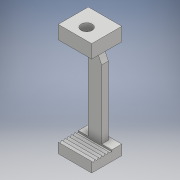
# Autodesk Inventor part: gravity-clamp-base5x5mm-part1-narrowTOP
Saved by Autodesk Inventor 2017 (Build 210142000, 142)
## iProperties
Created: 2021-08-04
Part Number: gravity-clamp-base5x5mm-part1-narrowTOP
Material: Generic
Document SubType Name: Modeling
Designer: Nikita
Density: 1 g/cm^3
Appearance: Default
Author: Nikita
Autodesk Inventor part; units mm, degrees
ref_plane "YZ Plane" through (0, 0, 0) normal (1, 0, 0) x (0, 1, 0)
ref_plane "XZ Plane" through (0, 0, 0) normal (0, 1, 0) x (-1, 0, 0)
ref_plane "XY Plane" through (0, 0, 0) normal (0, 0, 1) x (1, 0, 0)
sketch "Sketch1" plane through (0, 0, 0) normal (0, 0, 1) x (1, 0, 0)
  line L0 (0, 0) -> (10, 0)
  line L1 (10, 0) -> (10, 9)
  line L2 (10, 9) -> (0, 9)
  line L3 (0, 9) -> (0, 0)
  point P0 (5, 9)
  dimension "d0" = 10
  dimension "d1" = 9
  constraints: 8 end point, 2 parallel, 1 horizontal, 1 midpoint, 1 perpendicular
  measures "d0" distance of L2.end L1.end
  measures "d1" distance of L1.end L0.end
extrude "Extrusion1" add sketch "Sketch1" along normal blind 3
sketch "Sketch2" plane through (0, 0, 3) normal (0, 0, 1) x (1, 0, 0)
  line L0 (10, 9) -> (0, 9) projected
  circle A0 centre (5, 7) radius 1
  line L1 (0, 9) -> (0, 0) projected
  point P0 (5, 9)
  dimension "d4" = 2
  dimension "d5" = 2
  dimension "d67" = 5
  constraints: 1 centre point, 1 midpoint
  measures "d4" diameter of A0
  measures "d5" distance from line of A0.centre L0
  measures "d67" distance from line of L1 A0.centre
extrude "Extrusion2" add sketch "Sketch2" along normal blind 1.5
sketch "Sketch6" plane through (5, 7, 4.5) normal (0, 0, 1) x (1, 0, 0)
  circle A0 centre (0, 0) radius 1 projected
  line L0 (2, -1) -> (-2, -1)
  line L1 (-2, -1) -> (-2, 1)
  line L2 (-2, 1) -> (2, 1)
  line L3 (2, 1) -> (2, -1)
  line L4 (2, -1) -> (-2, 1) construction
  line L5 (-2, -1) -> (2, 1) construction
  point P0 (-5, -7)
  dimension "d13" = 4
  constraints: 12 end point, 2 midpoint, 2 parallel, 1 coincident, 1 horizontal, 1 perpendicular
  measures "d13" distance of L1.end L2.end
extrude "Extrusion5" add sketch "Sketch6" along normal blind 25
sketch "Sketch7" plane through (5, 7, 29.5) normal (0, 0, 1) x (1, 0, 0)
  circle A0 centre (0, 0) radius 1 projected
  line L0 (-5, -7) -> (5, -7) projected
  line L1 (5, -7) -> (5, 2) projected
  line L2 (5, 2) -> (-5, 2) projected
  line L3 (-5, 2) -> (-5, -7) projected
  arc A1 (0, -1) -> (0, 1) centre (0, 0) ccw projected
  arc A2 (0, 1) -> (0, -1) centre (0, 0) ccw projected
extrude "Extrusion6" add sketch "Sketch7" along normal blind 4 contours A0 | L3 L2 L1 L0
sketch "Sketch8" plane through (5, 7, 33.5) normal (0, 0, 1) x (1, 0, 0)
  line L0 (-5, -7) -> (5, -7) projected
  line L1 (5, -7) -> (5, 2) projected
  line L2 (5, 2) -> (-5, 2) projected
  line L3 (-5, 2) -> (-5, -7) projected
  circle A0 centre (0, -3.5) radius 1.65
  dimension "d18" = 3.3
  dimension "d66" = 5.5
  constraints: 1 centre point
  measures "d18" diameter of A0
  measures "d66" distance from line of A0.centre L2
extrude "Extrusion7" cut sketch "Sketch8" against normal blind 4 contours A0
sketch "Sketch10" plane through (0, 0, 0) normal (-1, 0, 0) x (0, 0, 1)
  line L0 (0, 0) -> (3, 0) projected
  line L1 (3, 0) -> (2.5, 0)
  line L2 (2.5, 0) -> (2.5, 0.5)
  line L3 (2.5, 6) -> (3, 6)
  line L4 (3, 6) -> (3, 5)
  line L5 (3, 0) -> (2.5, 0.5)
  line L6 (3, 0) -> (3.7071, 0) construction
  line L7 (2.5, 0.5) -> (3, 1)
  line L8 (3, 1) -> (2.5, 1.5)
  line L9 (2.5, 1.5) -> (3, 2)
  line L10 (3, 2) -> (2.5, 2.5)
  line L11 (2.5, 2.5) -> (3, 3)
  line L12 (3, 3) -> (2.5, 3.5)
  line L13 (2.5, 3.5) -> (3, 4)
  line L14 (3, 4) -> (2.5, 4.5)
  line L15 (2.5, 4.5) -> (3, 5)
  line L16 (3, 5) -> (2.5, 5.5)
  line L17 (2.5, 5.5) -> (3, 6)
  line L18 (2.5, 5.5) -> (2.5, 6)
  line L19 (2.5, 4.5) -> (2.5, 5.5)
  line L20 (2.5, 3.5) -> (2.5, 4.5)
  line L21 (2.5, 2.5) -> (2.5, 3.5)
  line L22 (2.5, 1.5) -> (2.5, 2.5)
  line L23 (2.5, 0.5) -> (2.5, 1.5)
  line L24 (3, 1) -> (3, 0)
  line L25 (3, 2) -> (3, 1)
  line L26 (3, 3) -> (3, 2)
  line L27 (3, 5) -> (3, 4)
  line L28 (3, 4) -> (3, 3)
  point P0 (2.5, 3)
  point P1 (3, 4.4114)
  point P2 (2.5, 4.5886)
  dimension "d23" = 0.5
  dimension "d24" = 6
  dimension "d25" = 135
  constraints: 56 end point, 43 parallel, 16 perpendicular, 2 horizontal, 2 point on line, 1 equal length
  measures "d23" distance of L3.start L3.end
  measures "d24" distance of L1.end L3.start
  measures "d25" angle of L6 L5
extrude "Extrusion10" add sketch "Sketch6" against normal up to surface (1.5 mm away) contours A0 L2 L3 L0 | A0 L0 L1 L2
sketch "Sketch12" plane through (5, 7, 29.5) normal (0, 0, -1) x (-1, 0, 0)
  circle A0 centre (0, 0) radius 1 projected
  line L0 (-2, 1) -> (-2, -1) projected
  line L1 (-2, -1) -> (2, -1) projected
  line L2 (2, 1) -> (-2, 1) projected
  line L3 (2, -1) -> (2, 1) projected
  point P0 (5, -7)
extrude "Extrusion11" cut sketch "Sketch12" along normal blind 4 contours A0 L2 L3 L1 | A0 L1 L0 L2
chamfer "Chamfer3" distance 2 distance2 1 1 edges at (3, 7, 25.5) measured on face at (3, 6.6667, 10.5)
chamfer "Chamfer4" distance 2 distance2 1 1 edges at (7, 7, 25.5) measured on face at (7, 7.3333, 10.5)
extrude "Extrusion12" cut sketch "Sketch10" against normal up to next contours L5 L7 L24 | L8 L9 L25 | L10 L11 L26 | L12 L13 L28 | L14 L15 L27 | L16 L17 L4 | L18 L3 L17
body "Solid1"
